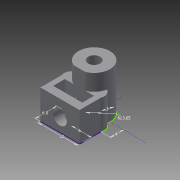
# Autodesk Inventor part: MotorAttachment2
Saved by Autodesk Inventor 2014 SP1 (Build 180222100, 222)
## iProperties
Created: 2015-03-26
Part Number: MotorAttachment2
Material: Generic
Document SubType Name: Modeling
Designer: Erin
Density: 1 g/cm^3
Appearance: Default
Author: Erin
Autodesk Inventor part; units mm, degrees
ref_plane "YZ Plane" through (0, 0, 0) normal (1, 0, 0) x (0, 1, 0)
ref_plane "XY Plane" through (0, 0, 0) normal (0, 0, 1) x (1, 0, 0)
sketch "Sketch1" plane through (0, 0, 0) normal (0, 0, 1) x (1, 0, 0)
  circle A0 centre (0, 0) radius 1.825
  circle A1 centre (0, 0) radius 4.825
  line L0 (-6, -4) -> (6, -4)
  line L1 (6, -10.5) -> (-6, -10.5)
  line L2 (-6, -10.5) -> (-6, -4)
  arc A2 (-2.3662, -0.949) -> (-6, -4) centre (-3.6609, -3.0965) ccw
  arc A3 (6, -4) -> (2.3662, -0.949) centre (3.6609, -3.0965) ccw
  arc A4 (-2.3662, -0.949) -> (2.3662, -0.949) centre (0, 0.4878) ccw
  line L3 (-15.4666, 0) -> (16.043, 0) construction
  line L4 (0, 8.2762) -> (0, -10.4238) construction
  line L5 (6, -10.5) -> (6, -4)
  dimension "d0" = 3.65
  dimension "d1" = 3
  dimension "d3" = 12
  dimension "d5" = 4
  dimension "d6" = 6.5
  dimension "d7" = 6
  constraints: 12 end point, 6 point on circle, 5 centre point, 2 horizontal, 2 parallel, 2 perpendicular, 1 coincident, 1 vertical
  measures "d0" diameter of A0
  measures "d1" radial gap between concentric circles of A0 A1
  measures "d3" distance of L1.start L1.end
  measures "d5" distance between parallel lines of L3 L0
  measures "d6" distance of L1.end L0.start
  measures "d7" distance between parallel lines of L4 L5
extrude "Extrusion1" add sketch "Sketch1" along normal blind 9
ref_plane "Work Plane1" through (0, -10.5, 0) normal (0, 1, 0) x (-1, 0, 0)
extrude "Extrusion4" add sketch "Sketch1" along normal blind 14 contours A1 A3 A4 A2 | A2 A4 A3 A1 L0 | L0 A1
sketch "Sketch2" plane through (0, -10.5, 0) normal (0, 1, 0) x (-1, 0, 0)
  line L0 (6, 0) -> (-6, 0) projected
  line L1 (-6, 0) -> (-6, 9) projected
  line L2 (6, 9) -> (-6, 9) projected
  line L3 (6, 0) -> (6, 9) projected
  circle A0 centre (0, 4) radius 2.125
  point P0 (0, 0)
  dimension "d11" = 4.25
  dimension "d12" = 4
  constraints: 1 centre point
  measures "d11" diameter of A0
  measures "d12" distance from line of L0 A0.centre
extrude "Extrusion2" cut sketch "Sketch2" along normal blind 8 contours A0
sketch "Sketch3" plane through (0, 0, 9) normal (0, 0, 1) x (1, 0, 0)
  line L0 (-6, -10.5) -> (6, -10.5) projected
  circle A0 centre (0, 0) radius 1.825 projected
  line L1 (-4.45, -4.5) -> (4.45, -4.5)
  line L2 (4.45, -4.5) -> (4.45, -8.1)
  line L3 (4.45, -8.1) -> (-4.45, -8.1)
  line L4 (-4.45, -8.1) -> (-4.45, -4.5)
  point P0 (0, -8.1)
  point P1 (0, -10.5)
  dimension "d15" = 8.9
  dimension "d16" = 3.6
  dimension "d17" = 4.5
  constraints: 8 end point, 2 midpoint, 2 parallel, 1 horizontal, 1 perpendicular, 1 vertical alignment
  measures "d15" distance of L2.end L3.end
  measures "d16" distance of L1.end L2.end
  measures "d17" distance from line of L1 A0.centre
extrude "Extrusion3" cut sketch "Sketch3" along normal mid plane 30 contours L1 L2 L3 L4
equation "\"d4\" = 0.4"
body "Solid1"
